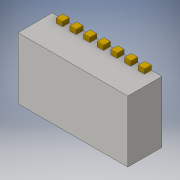
# Autodesk Inventor part: MC_BK377
Saved by Autodesk Inventor 2016 (Build 200138000, 138)
## iProperties
Created: 2016-08-30
Part Number: MC_BK377
Material: Generic
Document SubType Name: Modeling
Designer: jfixelle
Density: 1 g/cm^3
Appearance: Default
Author: jfixelle
Autodesk Inventor part; units mm, degrees
ref_plane "YZ Plane" through (0, 0, 0) normal (1, 0, 0) x (0, 1, 0)
ref_plane "XZ Plane" through (0, 0, 0) normal (0, 1, 0) x (-1, 0, 0)
ref_plane "XY Plane" through (0, 0, 0) normal (0, 0, 1) x (1, 0, 0)
sketch "Sketch1" plane through (0, 0, 0) normal (0, 0, 1) x (1, 0, 0)
  line L0 (-10.2, 5.715) -> (10.2, 5.715)
  line L1 (10.2, 5.715) -> (10.2, -5.715)
  line L2 (10.2, -5.715) -> (-10.2, -5.715)
  line L3 (-10.2, -5.715) -> (-10.2, 5.715)
  point P0 (0, 0)
  dimension "d0" = 20.4
  dimension "d1" = 10.2
  dimension "d2" = 11.43
  dimension "d3" = 5.715
  constraints: 8 end point, 2 parallel, 1 horizontal, 1 perpendicular
  measures "d0" distance of L0.start L0.end
  measures "d1" distance from line of point (0, 0) L1
  measures "d2" distance of L0.end L1.end
  measures "d3" distance from line of point (0, 0) L0
extrude "Extrusion1" add sketch "Sketch1" along normal blind 6.35
sketch "Sketch2" plane through (0, 0, 0) normal (0, 0, -1) x (-1, 0, 0)
  line L0 (8.205, 6.54) -> (7.015, 6.54)
  line L1 (7.015, 6.54) -> (7.015, 4.89)
  line L2 (7.015, 4.89) -> (8.205, 4.89)
  line L3 (8.205, 4.89) -> (8.205, 6.54)
  line L4 (10.2, 5.715) -> (-10.2, 5.715) projected
  line L5 (10.2, -5.715) -> (10.2, 5.715) projected
  point P0 (0, 0)
  dimension "d6" = 1.65
  dimension "d7" = 0.825
  dimension "d8" = 1.19
  dimension "d9" = 1.995
  constraints: 8 end point, 2 parallel, 1 horizontal, 1 perpendicular
  measures "d6" distance of L0.end L1.end
  measures "d7" distance between parallel lines of L0 L4
  measures "d8" distance of L0.start L0.end
  measures "d9" distance between parallel lines of L3 L5
extrude "Extrusion2" add sketch "Sketch2" against normal blind 1.27
pattern_linear "Rectangular Pattern1" count 7 spacing 2.54 along (1, 0, 0) of "Extrusion2"
mirror "Mirror1" about plane through (0, 0, 0) normal (0, 1, 0) of "Extrusion2", "Rectangular Pattern1"
body "Solid1"
